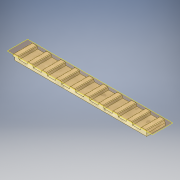
# Autodesk Inventor part: Large_Belt
Saved by Autodesk Inventor 2019.4 (Build 234330000, 330)
## iProperties
Created: 2021-02-02
Part Number: Large_Belt
Material: Rubber, Silicone
Document SubType Name: Modeling
Designer: Jorian Brusind
Density: 1.25 g/cm^3
Appearance: Fine - Cream
Author: Jorian Brusind
Autodesk Inventor part; units mm, degrees
ref_plane "YZ Plane" through (0, 0, 0) normal (1, 0, 0) x (0, 1, 0)
ref_plane "XZ Plane" through (0, 0, 0) normal (0, 1, 0) x (-1, 0, 0)
ref_plane "XY Plane" through (0, 0, 0) normal (0, 0, 1) x (1, 0, 0)
sketch "Sketch1" plane through (0, 0, 0) normal (0, 1, 0) x (-1, 0, 0)
  line L0 (0, 0) -> (100, 0)
  line L1 (100, 0) -> (100, -14)
  line L2 (100, -14) -> (0, -14)
  line L3 (0, -14) -> (0, 0)
  dimension "d0" = 100
  dimension "d1" = 14
  constraints: 8 end point, 2 parallel, 1 horizontal, 1 perpendicular
  measures "d0" distance of L1.end L2.end
  measures "d1" distance of L0.end L1.end
extrude "Extrusion1" add sketch "Sketch1" along normal blind 2
sketch "Sketch2" plane through (0, 2, 0) normal (0, 1, 0) x (1, 0, 0)
  line L0 (0, 0) -> (-4.75, 0)
  line L1 (-4.75, 0) -> (-4.75, 14)
  line L2 (-4.75, 14) -> (0, 14)
  line L3 (0, 14) -> (0, 0)
  dimension "d4" = 4.75
  dimension "d5" = 14
  constraints: 8 end point, 2 parallel, 1 horizontal, 1 perpendicular
  measures "d4" distance of L1.end L2.end
  measures "d5" distance of L0.end L1.end
ref_plane "Work Plane1" through (0, 4, 0) normal (0, 1, 0) x (1, 0, 0)
sketch "Sketch3" plane through (0, 4, 0) normal (0, 1, 0) x (1, 0, 0)
  line L0 (0, 0) -> (-0.5, 0)
  line L1 (-100, 0) -> (0, 0) projected
  line L2 (-0.5, 0) -> (-4.25, 0)
  line L3 (-4.25, 0) -> (-4.25, 14)
  line L4 (-4.25, 14) -> (-0.5, 14)
  line L5 (-0.5, 14) -> (-0.5, 0)
  dimension "d7" = 0.5
  dimension "d8" = 3.75
  dimension "d9" = 14
  constraints: 10 end point, 2 parallel, 1 horizontal, 1 perpendicular, 1 point on line
  measures "d7" distance of L0.start L0.end
  measures "d8" distance of L3.end L4.end
  measures "d9" distance of L2.end L3.end
loft "Loft1" add profiles "Sketch2", "Sketch3"
fillet "Fillet1" radius 0.5 2 edges at (-0.5, 4, -7) (-4.25, 4, -7)
pattern_linear "Rectangular Pattern2" count 10 spacing 10.75 along (-1, 0, 0) of "Loft1", "Fillet1"
body "Solid1"
